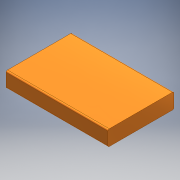
# Autodesk Inventor part: battery_40mah
Saved by Autodesk Inventor 2016 (Build 200138000, 138)
## iProperties
Created: 2016-08-08
Part Number: battery_40mah
Material: Gold
Document SubType Name: Modeling
Designer: rawrdong
Density: 19.3 g/cm^3
Appearance: Metal 1600F Hot
Author: rawrdong
Autodesk Inventor part; units mm, degrees
ref_plane "YZ Plane" through (0, 0, 0) normal (1, 0, 0) x (0, 1, 0)
ref_plane "XZ Plane" through (0, 0, 0) normal (0, 1, 0) x (-1, 0, 0)
ref_plane "XY Plane" through (0, 0, 0) normal (0, 0, 1) x (1, 0, 0)
sketch "Sketch1" plane through (0, 0, 0) normal (0, 0, 1) x (1, 0, 0)
  line L0 (-18.5, -12) -> (18.5, -12)
  line L1 (18.5, -12) -> (18.5, 12)
  line L2 (18.5, 12) -> (-18.5, 12)
  line L3 (-18.5, 12) -> (-18.5, -12)
  line L4 (-18.5, -12) -> (18.5, 12) construction
  line L5 (18.5, -12) -> (-18.5, 12) construction
  point P0 (0, 0)
  dimension "d0" = 24
  dimension "d1" = 37
  constraints: 12 end point, 2 midpoint, 2 parallel, 1 horizontal, 1 perpendicular
  measures "d0" distance of L0.end L1.end
  measures "d1" distance of L1.end L2.end
extrude "Extrusion1" add sketch "Sketch1" along normal blind 5.6
fillet "Fillet1" radius 0.5 4 edges at (0, 12, 5.6) (0, 12, 0) (0, -12, 5.6) (0, -12, 0)
body "Solid1"
